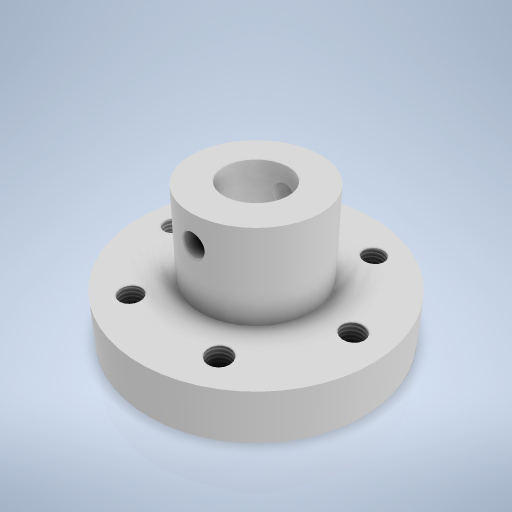
# Autodesk Inventor part: cover
Saved by Autodesk Inventor 2024.2 (Build 282272000, 272)
## iProperties
Created: 2024-05-05
Part Number: cover
Material: Generisch
Document SubType Name: Modeling
Designer: Fabri
Density: 1 g/cm^3
Appearance: Vorgabe
Author: Fabri
Autodesk Inventor part; units mm, degrees
ref_plane "YZ Plane" through (0, 0, 0) normal (1, 0, 0) x (0, 1, 0)
ref_plane "XY Plane" through (0, 0, 0) normal (0, 0, 1) x (1, 0, 0)
sketch "Skizze1" plane through (0, 0, 0) normal (0, 1, 0) x (-1, 0, 0)
  line L0 (0, 0) -> (28, 0)
  line L1 (28, 0) -> (28, -38)
  line L2 (28, -38) -> (58, -38)
  line L3 (58, -38) -> (58, -60)
  line L4 (58, -60) -> (0, -60)
  line L5 (0, -60) -> (0, 0)
  dimension "d0" = 116
  dimension "d1" = 56
  dimension "d2" = 22
  dimension "d3" = 38
  constraints: 12 end point, 5 perpendicular, 1 horizontal
  measures "d0" diameter of L3 L5
  measures "d1" diameter of L1 L5
  measures "d2" distance between parallel lines of L4 L2
  measures "d3" distance between parallel lines of L2 L0
revolve "Umdrehung1" add sketch "Skizze1" angle 360 about axis through (0, 0, -60) along (0, 0, 1)
sketch "Skizze2" plane through (0, 0, 0) normal (0, 0, 1) x (1, 0, 0)
  circle A0 centre (0, 0) radius 14
  dimension "d5" = 28
  constraints: 1 centre point, 1 coincident
  measures "d5" diameter of A0
extrude "Extrusion1" cut sketch "Skizze2" against normal up to surface (60 mm away)
ref_plane "Arbeitsebene1" through (0, 28, 0) normal (0, 1, 0) x (-1, 0, 0)
sketch "Skizze3" plane through (0, 28, 0) normal (0, 1, 0) x (-1, 0, 0)
  point P0 (0, 0)
  point P1 (0, -12)
  dimension "d9" = 12
  constraints: 1 vertical alignment
  measures "d9" distance of point (0, 0) point (0, -12)
hole "Bohrung1" at (0, 28, -12) direction (0, -1, 0) diameter 10 end through all
sketch "Skizze4" plane through (0, 0, -60) normal (0, 0, -1) x (-1, 0, 0)
  circle A0 centre (0, 0) radius 44 construction
  circle A1 centre (0, 0) radius 14 projected
  line L0 (0, 0) -> (0, 62.7079) construction
  line L1 (0, 0) -> (-33.1711, 57.4541) construction
  line L2 (0, 0) -> (35.197, 60.963) construction
  point P0 (-22, 38.1051)
  point P1 (22, 38.1051)
  dimension "d17" = 88
  dimension "d18" = 30
  dimension "d19" = 30
  constraints: 6 end point, 2 point on circle, 2 point on line, 1 centre point, 1 coincident, 1 vertical
  measures "d17" diameter of A0
  measures "d18" angle of L2 L0
  measures "d19" angle of L0 L1
hole "Bohrung2" at (22, 38.1051, -60) at (-22, 38.1051, -60) direction (0, 0, 1) diameter 10.106 depth 22 thread size "M12x1.75" class "6H" standard "ISO Metric profile"
pattern_circular "Runde Anordnung1" count 6 over 360 about axis through (0, 0, -49) along (0, 0, 1) of "Bohrung2"
